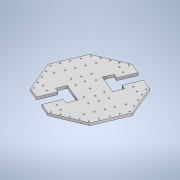
# Autodesk Inventor part: Support bas
Saved by Autodesk Inventor 2020 (Build 240168000, 168)
## iProperties
Created: 2019-11-28
Part Number: Support bas
Material: Générique
Document SubType Name: Modeling
Designer: erwan
Density: 1 g/cm^3
Appearance: Par défaut
Author: erwan
Autodesk Inventor part; units mm, degrees
ref_plane "YZ Plane" through (0, 0, 0) normal (1, 0, 0) x (0, 1, 0)
ref_plane "XZ Plane" through (0, 0, 0) normal (0, 1, 0) x (-1, 0, 0)
ref_plane "XY Plane" through (0, 0, 0) normal (0, 0, 1) x (1, 0, 0)
sketch "Esquisse1" plane through (0, 0, 0) normal (0, 1, 0) x (-1, 0, 0)
  line L0 (175, 0) -> (123.7437, 123.7437)
  line L1 (175, 0) -> (123.7437, -123.7437)
  line L2 (123.7437, -123.7437) -> (0, -175)
  line L3 (-123.7437, -123.7437) -> (-175, 0)
  line L4 (-175, 0) -> (-123.7437, 123.7437)
  line L5 (-123.7437, 123.7437) -> (0, 175)
  line L6 (-16.9098, -94.393) -> (-42.9323, -157.2169)
  line L7 (-54.7889, -78.703) -> (-80.8114, -141.5268)
  line L8 (-21.3074, -51.4406) -> (-58.2626, -36.1333)
  line L9 (16.9098, 94.393) -> (42.9323, 157.2169)
  line L10 (54.7889, 78.703) -> (80.8114, 141.5268)
  line L11 (123.7437, 123.7437) -> (80.8114, 141.5268)
  line L12 (42.9323, 157.2169) -> (0, 175)
  line L13 (0, -175) -> (-42.9323, -157.2169)
  line L14 (-123.7437, -123.7437) -> (-80.8114, -141.5268)
  line L15 (-21.3074, -51.4406) -> (15.6478, -66.748)
  line L16 (15.6478, -66.748) -> (1.1058, -101.8554)
  line L17 (1.1058, -101.8554) -> (-16.9098, -94.393)
  line L18 (-58.2626, -36.1333) -> (-72.8046, -71.2407)
  line L19 (-72.8046, -71.2407) -> (-54.7889, -78.703)
  line L20 (21.3074, 51.4406) -> (-15.6478, 66.748)
  line L21 (21.3074, 51.4406) -> (58.2626, 36.1333)
  line L22 (58.2626, 36.1333) -> (72.8046, 71.2407)
  line L23 (72.8046, 71.2407) -> (54.7889, 78.703)
  line L24 (-15.6478, 66.748) -> (-1.1058, 101.8554)
  line L25 (-1.1058, 101.8554) -> (16.9098, 94.393)
  point P0 (0, 0)
  constraints: 52 end point, 8 perpendicular, 1 collinear, 1 point on line
extrude "Extrusion1" add sketch "Esquisse1" along normal blind 10
sketch "Esquisse2" plane through (0, 10, 0) normal (0, 1, 0) x (1, 0, 0)
  line L0 (0, 0) -> (135.5137, -56.1316) construction
  line L1 (0, 0) -> (-162.1857, 67.1795) construction
  line L2 (0, 175) -> (-123.7437, -123.7437) construction
  line L3 (0, -175) -> (123.7437, 123.7437) construction
  line L4 (175, 0) -> (-123.7437, 123.7437) construction
  line L5 (-175, 0) -> (123.7437, -123.7437) construction
  line L6 (149.3718, 61.8718) -> (-149.3718, -61.8718) construction
  line L7 (-61.8718, 149.3718) -> (61.8718, -149.3718) construction
  line L8 (-61.8718, 149.3718) -> (-149.3718, -61.8718) construction
  line L9 (61.8718, -149.3718) -> (149.3718, 61.8718) construction
  circle A0 centre (165, 0) radius 2.25
  line L10 (165, 0) -> (115.2082, -120.2082) construction
  circle A1 centre (115.2082, -120.2082) radius 2.25
  circle A2 centre (140.8363, -58.3363) radius 2.25
  circle A3 centre (152.9182, -29.1682) radius 2.25
  circle A4 centre (128.0222, -89.2722) radius 2.25
  line L11 (119.9169, 114.5049) -> (165, 0) construction
  circle A5 centre (119.9169, 114.5049) radius 2.25
  circle A6 centre (141.8641, 58.762) radius 2.25
  circle A7 centre (130.8905, 86.6335) radius 2.25
  circle A8 centre (153.432, 29.381) radius 2.25
  line L12 (3.8268, -165.7612) -> (115.2082, -120.2082) construction
  circle A9 centre (3.8268, -165.7612) radius 2.25
  circle A10 centre (59.5175, -142.9847) radius 2.25
  circle A11 centre (31.6722, -154.3729) radius 2.25
  circle A12 centre (87.3628, -131.5964) radius 2.25
  line L13 (-165, 0) -> (-115.2082, 120.2082) construction
  circle A13 centre (-165, 0) radius 2.25
  circle A14 centre (-115.2082, 120.2082) radius 2.25
  circle A15 centre (-140.8363, 58.3363) radius 2.25
  circle A16 centre (-128.0222, 89.2722) radius 2.25
  circle A17 centre (-152.9182, 29.1682) radius 2.25
  line L14 (-3.8268, 165.7612) -> (-115.2082, 120.2082) construction
  circle A18 centre (-3.8268, 165.7612) radius 2.25
  circle A19 centre (-59.2684, 143.0866) radius 2.25
  circle A20 centre (-31.6722, 154.3729) radius 2.25
  circle A21 centre (-87.3628, 131.5964) radius 2.25
  line L15 (-119.9169, -114.5049) -> (-165, 0) construction
  circle A22 centre (-119.9169, -114.5049) radius 2.25
  circle A23 centre (-141.8641, -58.762) radius 2.25
  circle A24 centre (-130.8905, -86.6335) radius 2.25
  circle A25 centre (-153.432, -29.381) radius 2.25
  circle A26 centre (15.3073, -138.0448) radius 2.25
  circle A27 centre (79.9937, -105.6218) radius 2.25
  circle A28 centre (105.6218, -43.75) radius 2.25
  circle A29 centre (131.25, 18.1218) radius 2.25
  circle A30 centre (108.4363, 86.7885) radius 2.25
  circle A31 centre (61.8718, -25.6282) radius 2.25
  circle A32 centre (0, 0) radius 2.25
  circle A33 centre (-15.3073, 138.0448) radius 2.25
  circle A34 centre (-79.9937, 105.6218) radius 2.25
  circle A35 centre (-105.6218, 43.75) radius 2.25
  circle A36 centre (-131.25, -18.1218) radius 2.25
  circle A37 centre (-61.8718, 25.6282) radius 2.25
  line L16 (183.0548, 10.7676) -> (-121.8254, 137.0531) construction
  line L17 (-121.8254, 137.0531) -> (-183.0548, -10.7676) construction
  line L18 (-183.0548, -10.7676) -> (121.8254, -137.0531) construction
  line L19 (183.0548, 10.7676) -> (121.8254, -137.0531) construction
  line L20 (-52.2625, 153.3522) -> (145.3915, 71.4812) construction
  line L21 (15.3073, -138.0448) -> (-145.3915, -71.4812) construction
  line L22 (15.3073, -138.0448) -> (52.2625, -153.3522) construction
  circle A38 centre (-108.4363, -86.7885) radius 2.25
  line L23 (72.8046, 71.2407) -> (99.3535, 133.8464) construction
  line L24 (-1.1058, 101.8554) -> (25.4432, 164.4611) construction
  line L25 (1.1058, -101.8554) -> (-25.4432, -164.4611) construction
  line L26 (-72.8046, -71.2407) -> (-98.8273, -134.0651) construction
  line L27 (-15.6478, 66.748) -> (-57.8915, -35.2375) construction
  line L28 (58.2626, 36.1333) -> (15.8255, -66.3188) construction
  circle A39 centre (-9.8261, -127.6342) radius 2.25
  circle A40 centre (-83.5197, -97.1093) radius 2.25
  circle A41 centre (37.0441, -15.0928) radius 2.25
  circle A42 centre (-36.7697, 15.7552) radius 2.25
  line L29 (31.2572, -99.5385) -> (49.7348, -107.1922) construction
  line L30 (49.7348, -107.1922) -> (42.0811, -125.6698) construction
  line L31 (42.0811, -125.6698) -> (23.6035, -118.0161) construction
  line L32 (31.2572, -99.5385) -> (23.6035, -118.0161) construction
  line L33 (92.4865, 48.2822) -> (110.9641, 40.6285) construction
  line L34 (110.9641, 40.6285) -> (118.6178, 59.1061) construction
  line L35 (118.6178, 59.1061) -> (100.1402, 66.7598) construction
  line L36 (92.4865, 48.2822) -> (100.1402, 66.7598) construction
  line L37 (-92.4865, -48.2822) -> (-110.9641, -40.6285) construction
  line L38 (-110.9641, -40.6285) -> (-118.6178, -59.1061) construction
  line L39 (-118.6178, -59.1061) -> (-100.1402, -66.7598) construction
  line L40 (-92.4865, -48.2822) -> (-100.1402, -66.7598) construction
  line L41 (-31.2572, 99.5385) -> (-23.6035, 118.0161) construction
  line L42 (-23.6035, 118.0161) -> (-42.0811, 125.6698) construction
  line L43 (-42.0811, 125.6698) -> (-49.7348, 107.1922) construction
  line L44 (-31.2572, 99.5385) -> (-49.7348, 107.1922) construction
  line L45 (-152.9182, 29.1682) -> (128.0222, -89.2722) construction
  line L46 (152.9182, -29.1682) -> (-128.0222, 89.2722) construction
  circle A43 centre (-117.7952, 14.3608) radius 2.25
  circle A44 centre (-92.8993, 74.4649) radius 2.25
  circle A45 centre (117.7952, -14.3608) radius 2.25
  circle A46 centre (92.8993, -74.4649) radius 2.25
  circle A47 centre (49.263, -56.0685) radius 2.25
  circle A48 centre (-74.159, -4.0356) radius 2.25
  circle A49 centre (-49.263, 56.0685) radius 2.25
  circle A50 centre (74.159, 4.0356) radius 2.25
  circle A51 centre (-42.2349, -17.4943) radius 2.25
  circle A52 centre (-17.7153, 42.7684) radius 2.25
  circle A53 centre (42.2349, 17.4943) radius 2.25
  circle A54 centre (17.7153, -42.7684) radius 2.25
  circle A55 centre (9.8261, 127.6342) radius 2.25
  circle A56 centre (83.7365, 97.0195) radius 2.25
  dimension "d14" = 4.5
  dimension "d15" = 4.5
  dimension "d16" = 4.5
  dimension "d17" = 4.5
  dimension "d18" = 4.5
  dimension "d19" = 10
  dimension "d20" = 4.5
  dimension "d21" = 4.5
  dimension "d22" = 4.5
  dimension "d23" = 4.5
  dimension "d24" = 10
  dimension "d25" = 4.5
  dimension "d26" = 4.5
  dimension "d27" = 4.5
  dimension "d28" = 4.5
  dimension "d29" = 10
  dimension "d30" = 4.5
  dimension "d31" = 4.5
  dimension "d32" = 4.5
  dimension "d33" = 4.5
  dimension "d34" = 4.5
  dimension "d35" = 10
  dimension "d36" = 4.5
  dimension "d37" = 4.5
  dimension "d38" = 4.5
  dimension "d39" = 4.5
  dimension "d40" = 10
  dimension "d41" = 4.5
  dimension "d42" = 4.5
  dimension "d43" = 4.5
  dimension "d44" = 4.5
  dimension "d45" = 4.5
  dimension "d46" = 4.5
  dimension "d47" = 4.5
  dimension "d48" = 4.5
  dimension "d49" = 4.5
  dimension "d51" = 4.5
  dimension "d53" = 4.5
  dimension "d54" = 4.5
  dimension "d56" = 4.5
  dimension "d57" = 4.5
  dimension "d58" = 4.5
  dimension "d60" = 4.5
  dimension "d68" = 330
  dimension "d69" = 160
  dimension "d82" = 4.5
  dimension "d83" = 4.5
  dimension "d84" = 4.5
  dimension "d85" = 4.5
  dimension "d86" = 4.5
  dimension "d87" = 20
  dimension "d88" = 20
  dimension "d89" = 20
  dimension "d90" = 20
  dimension "d91" = 20
  dimension "d92" = 20
  dimension "d93" = 20
  dimension "d94" = 20
  dimension "d95" = 4.5
  dimension "d96" = 4.5
  dimension "d97" = 4.5
  dimension "d98" = 4.5
  dimension "d99" = 4.5
  dimension "d100" = 4.5
  constraints: 90 end point, 60 point on line, 57 centre point, 9 perpendicular, 8 coincident, 5 midpoint, 3 parallel, 1 collinear, 32 other
  measures "d14" diameter of A0
  measures "d15" diameter of A1
  measures "d16" diameter of A2
  measures "d17" diameter of A3
  measures "d18" diameter of A4
  measures "d19" distance of point (123.744, 123.744) L11.start
  measures "d20" diameter of A5
  measures "d21" diameter of A6
  measures "d22" diameter of A7
  measures "d23" diameter of A8
  measures "d24" distance of point (0, -175) L12.start
  measures "d25" diameter of A9
  measures "d26" diameter of A10
  measures "d27" diameter of A11
  measures "d28" diameter of A12
  measures "d29" distance of L5.start L13.start
  measures "d30" diameter of A13
  measures "d31" diameter of A14
  measures "d32" diameter of A15
  measures "d33" diameter of A16
  measures "d34" diameter of A17
  measures "d35" distance of point (0, 175) L14.start
  measures "d36" diameter of A18
  measures "d37" diameter of A19
  measures "d38" diameter of A20
  measures "d39" diameter of A21
  measures "d40" distance of point (-123.744, -123.744) L15.start
  measures "d41" diameter of A22
  measures "d42" diameter of A23
  measures "d43" diameter of A24
  measures "d44" diameter of A25
  measures "d45" diameter of A26
  measures "d46" diameter of A27
  measures "d47" diameter of A28
  measures "d48" diameter of A29
  measures "d49" diameter of A30
  measures "d51" diameter of A31
  measures "d53" diameter of A32
  measures "d54" diameter of A33
  measures "d56" diameter of A34
  measures "d57" diameter of A35
  measures "d58" diameter of A36
  measures "d60" diameter of A37
  measures "d68" distance of L16.start L16.end
  measures "d69" distance of L16.end L17.end
  measures "d82" diameter of A38
  measures "d83" diameter of A39
  measures "d84" diameter of A40
  measures "d85" diameter of A41
  measures "d86" diameter of A42
  measures "d87" distance of L29.start L29.end
  measures "d88" distance of L29.end L30.end
  measures "d89" distance of L33.start L33.end
  measures "d90" distance of L33.end L34.end
  measures "d91" distance of L37.start L37.end
  measures "d92" distance of L37.end L38.end
  measures "d93" distance of L41.start L41.end
  measures "d94" distance of L41.end L42.end
  measures "d95" diameter of A43
  measures "d96" diameter of A44
  measures "d97" diameter of A45
  measures "d98" diameter of A46
  measures "d99" diameter of A47
  measures "d100" diameter of A48
extrude "Extrusion2" cut sketch "Esquisse2" against normal blind 10
